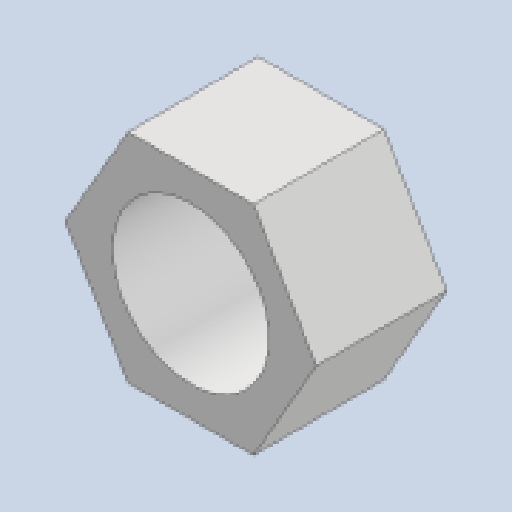
# Autodesk Inventor part: 너트6
Saved by Autodesk Inventor 2023.1 (Build 271208000, 208)
## iProperties
Created: 2022-10-19
Part Number: 너트6
Material: 철, 회색
Document SubType Name: Modeling
Designer: PARK
Density: 7.15 g/cm^3
Appearance: 철 회색
Author: PARK
Autodesk Inventor part; units mm, degrees
ref_plane "YZ Plane" through (0, 0, 0) normal (1, 0, 0) x (0, 1, 0)
ref_plane "XZ Plane" through (0, 0, 0) normal (0, 1, 0) x (-1, 0, 0)
ref_plane "XY Plane" through (0, 0, 0) normal (0, 0, 1) x (1, 0, 0)
sketch "스케치1" plane through (0, 0, 0) normal (0, 0, 1) x (1, 0, 0)
  circle A0 centre (0, 0) radius 3
  line L0 (-4.809, 0) -> (-2.4045, 4.1647)
  line L1 (-2.4045, 4.1647) -> (2.4045, 4.1647)
  line L2 (2.4045, 4.1647) -> (4.809, 0)
  line L3 (4.809, 0) -> (2.4045, -4.1647)
  line L4 (2.4045, -4.1647) -> (-2.4045, -4.1647)
  line L5 (-2.4045, -4.1647) -> (-4.809, 0)
  dimension "d0" = 6
  constraints: 12 end point, 1 centre point, 1 coincident, 13 other
  measures "d0" diameter of A0
extrude "돌출1" add sketch "스케치1" along normal blind 5
thread "스레드1" size "M6x1" class "6H" standard "ANSI Metric M Profile" full length
